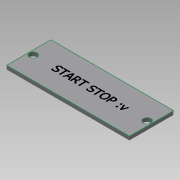
# Autodesk Inventor part: Start Stop
Saved by Autodesk Inventor 2015 SP1 (Build 190203100, 203)
## iProperties
Created: 2015-02-09
Part Number: Start Stop
Material: Generic
Document SubType Name: Modeling
Designer: Rafi Kurnia Putra
Density: 1 g/cm^3
Appearance: Default
Mass: 1.8485 g
Surface Area: 24.6858 cm^2
Volume: 1.8485 cm^3
Author: Rafi Kurnia Putra
Autodesk Inventor part; units mm, degrees
ref_plane "YZ Plane" through (0, 0, 0) normal (1, 0, 0) x (0, 1, 0)
ref_plane "XZ Plane" through (0, 0, 0) normal (0, 1, 0) x (-1, 0, 0)
ref_plane "XY Plane" through (0, 0, 0) normal (0, 0, 1) x (1, 0, 0)
sketch "Sketch1" plane through (0, 0, 0) normal (0, 1, 0) x (-1, 0, 0)
  line L0 (27.7495, 9.9695) -> (-27.7495, 9.9695)
  line L1 (-27.7495, 9.9695) -> (-27.7495, -9.9695)
  line L2 (-27.7495, -9.9695) -> (27.7495, -9.9695)
  line L3 (27.7495, -9.9695) -> (27.7495, 9.9695)
  line L4 (27.7495, 9.9695) -> (-27.7495, -9.9695) construction
  line L5 (-27.7495, 9.9695) -> (27.7495, -9.9695) construction
  circle A0 centre (25.7175, 0) radius 1.75
  circle A1 centre (-25.7175, 0) radius 1.75
  point P0 (0, 0)
  dimension "d0" = 55.499
  dimension "d1" = 19.939
  dimension "d2" = 3.5
  dimension "d3" = 3.5
  dimension "d4" = 2.032
  dimension "d5" = 2.032
  constraints: 12 end point, 2 centre point, 2 midpoint, 2 parallel, 1 horizontal, 1 perpendicular
  measures "d0" distance of L2.end L1.end
  measures "d1" distance of L1.end L0.end
  measures "d2" diameter of A0
  measures "d3" diameter of A1
  measures "d4" distance from line of A0.centre L3
  measures "d5" distance from line of A1.centre L1
extrude "Extrusion1" add sketch "Sketch1" along normal blind 1.7
sketch "Sketch2" plane through (0, 1.7, 0) normal (0, 1, 0) x (1, 0, 0)
  circle A0 centre (25.7175, 0) radius 1.75 projected
  circle A1 centre (-25.7175, 0) radius 1.75 projected
  line L0 (-27.7495, -9.9695) -> (27.7495, -9.9695) projected
  line L1 (27.7495, -9.9695) -> (27.7495, 9.9695) projected
  line L2 (27.7495, 9.9695) -> (-27.7495, 9.9695) projected
  line L3 (-27.7495, 9.9695) -> (-27.7495, -9.9695) projected
  line L4 (16.1881, -1.9444) -> (-16.645, -1.9444) construction
  line L5 (-16.645, -1.9444) -> (-16.645, 1.7031) construction
  line L6 (-16.645, 1.7031) -> (16.1881, 1.7031) construction
  line L7 (16.1881, 1.7031) -> (16.1881, -1.9444) construction
  point P0 (0, 0)
  constraints: 2 other
body "Solid1"
